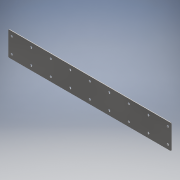
# Autodesk Inventor part: IMS-10-002
Saved by Autodesk Inventor 2021 (Build 250183000, 183)
## iProperties
Created: 2020-10-06
Part Number: IMS-10-002
Material: Steel, Carbon
Document SubType Name: Sheet Metal
Designer: mahra
Density: 7.85 g/cm^3
Sheet Metal Rule: Default_mm
Appearance: Semi-Polished
Mass: 2836.02 g
Surface Area: 1917.11 cm^2
Volume: 361.277 cm^3
Author: mahra
Autodesk Inventor part; units mm, degrees
ref_plane "YZ Plane" through (0, 0, 0) normal (1, 0, 0) x (0, 1, 0)
ref_plane "XZ Plane" through (0, 0, 0) normal (0, 1, 0) x (-1, 0, 0)
ref_plane "XY Plane" through (0, 0, 0) normal (0, 0, 1) x (1, 0, 0)
sketch "Sketch1" plane through (0, 0, 0) normal (0, 0, 1) x (1, 0, 0)
  line L0 (-417.5, 62.5) -> (417.5, 62.5)
  line L1 (417.5, 62.5) -> (417.5, -62.5)
  line L2 (417.5, -62.5) -> (-417.5, -62.5)
  line L3 (-417.5, -62.5) -> (-417.5, 62.5)
  line L4 (-417.5, 62.5) -> (417.5, -62.5) construction
  line L5 (417.5, 62.5) -> (-417.5, -62.5) construction
  point P0 (0, 0)
  dimension "d0" = 125
  dimension "d1" = 835
  measures "d0" distance of L2.end L0.start
  measures "d1" distance of L0.start L0.end
extrude "Plate1" add sketch "Sketch1" along normal blind 3
sketch "Sketch2" plane through (0, 0, 3) normal (0, 0, 1) x (1, 0, 0)
  circle A0 centre (0, 40) radius 5.35
  circle A1 centre (0, -40) radius 5.35
  line L0 (0, 40) -> (0, -40)
  point P0 (0, 0)
  point P1 (0, 0)
  dimension "d3" = 10.7
  dimension "d4" = 80
  constraints: 2 centre point, 2 end point, 2 vertical alignment, 1 coincident, 1 equal radius, 1 midpoint, 1 vertical
  measures "d3" diameter of A0
  measures "d4" distance of L0.start L0.end
extrude "Cut1" cut sketch "Sketch2" against normal blind 3
pattern_linear "Rectangular Pattern1" count 9 spacing 100 along (1, 0, 0) of "Cut1" first direction both ways yes
fillet "Fillet1" radius 5 4 edges at (417.5, -62.5, 1.5) (417.5, 62.5, 1.5) (-417.5, -62.5, 1.5) (-417.5, 62.5, 1.5)
equation "\"d5\" = Thickness"
equation "\"d2\" = Thickness"
equation "\"BendRadius\" = Thickness"
equation "\"BendReliefWidth\" = Thickness"
equation "\"BendReliefDepth\" = 0.5 * Thickness"
equation "\"CornerReliefSize\" = 4 * Thickness"
equation "\"MinimumRemnant\" = 2 * Thickness"
equation "\"TransitionRadius\" = BendRadius"
equation "\"JacobiRadiusSize\" = BendRadius"
equation "\"GapSize\" = Thickness"
equation "\"Thickness\" = 3"
body "Solid1"
